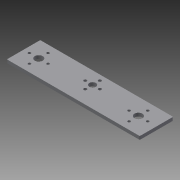
# Autodesk Inventor part: print bed test strut
Saved by Autodesk Inventor 2014 SP1 (Build 180222100, 222)
## iProperties
Created: 2014-11-30
Part Number: print bed test strut
Material: Generic
Document SubType Name: Modeling
Designer: Mon
Density: 1 g/cm^3
Appearance: Default
Author: Mon
Autodesk Inventor part; units mm, degrees
ref_plane "YZ Plane" through (0, 0, 0) normal (1, 0, 0) x (0, 1, 0)
ref_plane "XZ Plane" through (0, 0, 0) normal (0, 1, 0) x (-1, 0, 0)
ref_plane "XY Plane" through (0, 0, 0) normal (0, 0, 1) x (1, 0, 0)
sketch "Sketch1" plane through (0, 0, 0) normal (0, 0, 1) x (1, 0, 0)
  line L0 (199.9787, 50.2308) -> (-0.0213, 50.2308)
  circle A0 centre (172.7248, 39.2308) radius 2
  circle A1 centre (158.7248, 25.2308) radius 2
  circle A2 centre (172.7248, 11.2308) radius 2
  circle A3 centre (186.7248, 25.2308) radius 2
  circle A4 centre (22.7248, 39.2308) radius 2
  circle A5 centre (8.7248, 25.2308) radius 2
  circle A6 centre (22.7248, 11.2308) radius 2
  circle A7 centre (36.7248, 25.2308) radius 2
  circle A8 centre (97.7248, 31.2308) radius 5
  circle A9 centre (172.7248, 25.2308) radius 6
  circle A10 centre (22.7248, 25.2308) radius 6
  circle A11 centre (97.7248, 20.2308) radius 2.25
  circle A12 centre (86.7248, 31.2308) radius 2.25
  circle A13 centre (108.7248, 31.2308) radius 2.25
  circle A14 centre (97.7248, 42.2308) radius 2.25
  line L1 (-0.0213, 50.2308) -> (-0.0213, 0)
  line L2 (-0.0213, 0) -> (199.9787, 0)
  line L3 (199.9787, 0) -> (199.9787, 50.2308)
  point P0 (0, 0)
  constraints: 15 centre point, 8 end point
extrude "Extrusion1" add sketch "Sketch1" along normal blind 5
fillet "Fillet1" radius 1 1 edges at (199.9787, 50.2308, 2.5)
fillet "Fillet2" radius 1 1 edges at (199.9787, 0, 2.5)
fillet "Fillet3" radius 1 1 edges at (-0.0213, 0, 2.5)
fillet "Fillet4" radius 1 1 edges at (-0.0213, 50.2308, 2.5)
body "Solid1"
